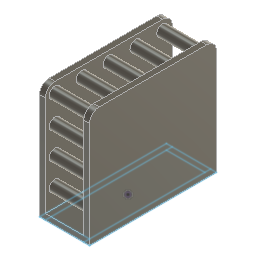
Странный но прикольный органайзер (Autodesk Fusion 360 design; units mm, degrees)
Autodesk Fusion 360 part; units mm, degrees
note: some values were not read from the file. Set by a fixed rule: which sketch regions a step uses.
sketch "Sketch1" plane through (0, 0, 0) normal (0, 0, 1) x (1, 0, 0)
  line L0 (10, -30) -> (-10, -30)
  line L1 (-10, -33) -> (-10, 33)
  line L2 (-10, 30) -> (10, 30)
  line L3 (10, 33) -> (10, -33)
  line L4 (-13, -33) -> (-13, 33)
  line L5 (-13, 33) -> (13, 33)
  line L6 (13, 33) -> (13, -33)
  line L7 (13, -33) -> (-13, -33)
  constraint horizontal L0
  constraint perpendicular L0 L1
  constraint parallel L0 L2
  constraint parallel L1 L3
  constraint coincident L5 L1.end
  constraint coincident L2.start L1
  constraint coincident L5 L3.start
  constraint coincident L2.end L3
  constraint coincident L7 L3.end
  constraint coincident L0.start L3
  constraint coincident L7 L1.start
  constraint coincident L0.end L1
extrude "Extrude1" add sketch "Sketch1" along normal blind 3
extrude "Extrude2" add sketch "Sketch1" along normal blind 60 contours L3 L5 L6 L7 | L1 L4 L5 L7
sketch "Sketch2" plane through (13, 0, 0) normal (1, 0, 0) x (0, 1, 0)
  line L0 (-33, 0) -> (33, 0)
  line L1 (33, 0) -> (33, 60)
  line L2 (33, 60) -> (-33, 60)
  line L3 (-33, 60) -> (-33, 0)
  circle A0 centre (-28, 55) radius 3
  circle A1 centre (0, 55) radius 3
  circle A2 centre (-14, 55) radius 3
  line L4 (0, 1.75) -> (0, 22.5)
  circle A3 centre (14, 55) radius 3
  circle A4 centre (28, 55) radius 3
  circle A5 centre (-28, 41) radius 3
  circle A6 centre (-14, 41) radius 3
  circle A7 centre (0, 41) radius 3
  circle A8 centre (14, 41) radius 3
  circle A9 centre (28, 41) radius 3
  circle A10 centre (-28, 27) radius 3
  circle A11 centre (-14, 27) radius 3
  circle A12 centre (0, 27) radius 3
  circle A13 centre (14, 27) radius 3
  circle A14 centre (28, 27) radius 3
  circle A15 centre (-28, 13) radius 3
  circle A16 centre (-14, 13) radius 3
  circle A17 centre (0, 13) radius 3
  circle A18 centre (14, 13) radius 3
  circle A19 centre (28, 13) radius 3
  dimension "d8" = 0
  dimension "d9" = -42
  constraint symmetric A0 L4 A4
  constraint symmetric A2 L4 A3
extrude "Extrude3" add sketch "Sketch2" against normal blind 26 contours A0 | A1 | A2 | L4 A17 | L4 A17 | A3 | A4 | A5 | A6 | A7 | A8 | A9 | A10 | A11 | A12 | A13 | A14 | A15 | A16 | A18 | A19
fillet "Fillet1" radius 5 4 edges at (11.5, -33, 60) (-11.5, -33, 60) (11.5, 33, 60) (-11.5, 33, 60)
